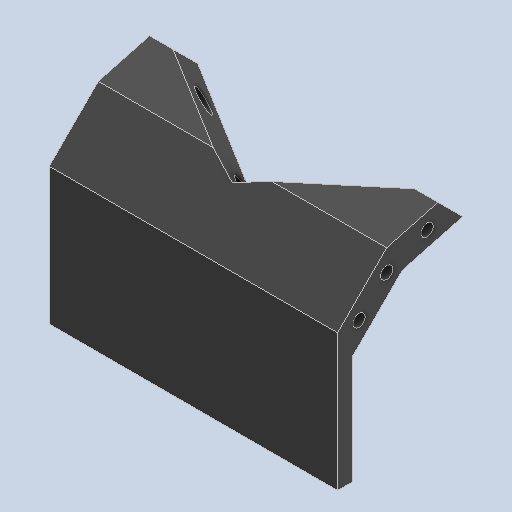
# Autodesk Inventor part: upper
Saved by Autodesk Inventor 2024.1 (Build 281209000, 209)
## iProperties
Created: 2024-10-11
Part Number: upper
Material: 一般
Document SubType Name: Modeling
Designer: hibik
Density: 1 g/cm^3
Appearance: 既定
Author: hibik
Autodesk Inventor part; units mm, degrees
ref_plane "YZ Plane" through (0, 0, 0) normal (1, 0, 0) x (0, 1, 0)
ref_plane "XZ Plane" through (0, 0, 0) normal (0, 1, 0) x (-1, 0, 0)
sketch "スケッチ1" plane through (0, 0, 0) normal (1, 0, 0) x (0, 1, 0)
  line L0 (0, 0) -> (18, 0)
  line L1 (18, 0) -> (18, -2)
  line L2 (18, -2) -> (0, -2)
  line L3 (0, -2) -> (0, 0)
  line L4 (18, 0) -> (39.2132, -21.2132)
  line L5 (39.2132, -21.2132) -> (37.799, -22.6274)
  line L6 (37.799, -22.6274) -> (17.1716, -2)
  dimension "d0" = 2
  dimension "d1" = 18
  dimension "d4" = 30
  dimension "d5" = 135
  dimension "d6" = 2
  constraints: 14 end point, 3 perpendicular, 2 parallel, 1 horizontal, 1 point on line
  measures "d0" distance of L0.end L1.end
  measures "d1" distance of L1.end L2.end
  measures "d4" distance from line of L0.end L5
  measures "d5" angle of L0 L4
  measures "d6" distance from line of L4.end L6
extrude "押し出し1" add sketch "スケッチ1" along normal blind 38
sketch "スケッチ2" plane through (38, 0, 0) normal (1, 0, 0) x (0, 0, -1)
  line L0 (13.2259, 26.2762) -> (6.4645, 24.4645) projected
  line L1 (2, 0) -> (2, 17.1716) projected
  line L2 (2, 17.1716) -> (22.6274, 37.799) projected
  line L3 (22.6274, 37.799) -> (21.2132, 39.2132) projected
  line L4 (21.2132, 39.2132) -> (0, 18) projected
  line L5 (0, 18) -> (0, 0) projected
  line L6 (0, 0) -> (2, 0) projected
  point P0 (10.3282, 25.4997)
extrude "押し出し2" cut sketch "スケッチ2" against normal through all contours L0 L4 L3 L2
sketch "スケッチ3" plane through (38, 0, 0) normal (1, 0, 0) x (0, 0, -1)
  line L0 (0, -0.1838) -> (49.5981, -49.7818) projected
  line L1 (49.5981, -49.7818) -> (50.9877, -48.3922) projected
  line L2 (50.9877, -48.3922) -> (50.3051, -40.5894) projected
  line L3 (50.3051, -40.5894) -> (38.2775, -28.5617) projected
  line L4 (38.2775, -28.5617) -> (34.3952, -14.0729) projected
  line L5 (34.3952, -14.0729) -> (39.6985, -8.7696) projected
  line L6 (25.2028, 5.7261) -> (39.6985, -8.7696) projected
  line L7 (25.2028, 9.9688) -> (25.2468, 10.0127) projected
  line L8 (25.2468, 14.2554) -> (13.2259, 26.2762) projected
  line L9 (13.2259, 26.2762) -> (6.4645, 24.4645) projected
  line L10 (6.4645, 24.4645) -> (0, 18) projected
  circle A0 centre (45.0018, -38.8216) radius 0.8 projected
  circle A1 centre (48.5373, -42.3571) radius 0.8 projected
  line L11 (25.2886, 2.8119) -> (28.6525, -0.552) projected
  arc A2 (29.0919, -1.6127) -> (28.6525, -0.552) centre (27.5919, -1.6127) ccw projected
  line L12 (29.0919, -1.6127) -> (29.0919, -20.7046) projected
  arc A3 (26.5312, -21.7652) -> (29.0919, -20.7046) centre (27.5919, -20.7046) ccw projected
  line L13 (26.5312, -21.7652) -> (23.1673, -18.4013) projected
  arc A4 (22.7279, -17.3406) -> (23.1673, -18.4013) centre (24.2279, -17.3406) ccw projected
  line L14 (22.7279, -17.3406) -> (22.7279, 1.7513) projected
  arc A5 (25.2886, 2.8119) -> (22.7279, 1.7513) centre (24.2279, 1.7513) ccw projected
  line L15 (13.8033, -9.0373) -> (10.4393, -5.6734) projected
  arc A6 (10, -4.6127) -> (10.4393, -5.6734) centre (11.5, -4.6127) ccw projected
  line L16 (10, -4.6127) -> (10, 14.4792) projected
  arc A7 (12.5607, 15.5398) -> (10, 14.4792) centre (11.5, 14.4792) ccw projected
  line L17 (12.5607, 15.5398) -> (15.9246, 12.1759) projected
  arc A8 (16.364, 11.1152) -> (15.9246, 12.1759) centre (14.864, 11.1152) ccw projected
  line L18 (16.364, 11.1152) -> (16.364, -7.9767) projected
  arc A9 (13.8033, -9.0373) -> (16.364, -7.9767) centre (14.864, -7.9767) ccw projected
  line L19 (2, 0) -> (2, 17.1716) projected
  line L20 (2, 14.3431) -> (13.5795, 25.9226)
  line L21 (16.4919, 23.0102) -> (8.535, 20.8782)
  line L22 (6.4645, 24.4645) -> (0, 18) projected
  line L23 (2, 17.1716) -> (10.3282, 25.4997) projected
  circle A10 centre (11.8117, 23.8267) radius 0.8 projected
  circle A11 centre (2.8284, 18) radius 0.8 projected
  circle A12 centre (6.4645, 21.636) radius 0.8 projected
  arc A13 (25.2028, 9.9688) -> (25.2028, 5.7261) centre (27.3241, 7.8475) ccw projected
  circle A14 centre (16.7615, 19.9122) radius 0.8 projected
  line L24 (0, 18) -> (0, -0.1838) projected
  arc A15 (25.2468, 10.0127) -> (25.2468, 14.2554) centre (23.1254, 12.1341) ccw projected
  circle A16 centre (20.297, 16.3767) radius 0.8 projected
  point P0 (0, 0)
  dimension "d9" = 4
  dimension "d10" = 4
  constraints: 4 end point, 4 point on line, 2 parallel, 1 perpendicular
  measures "d9" distance between parallel lines of L10 L20
  measures "d10" distance between parallel lines of L9 L21
ref_plane "作業平面1" through (0, -49.7818, -69.441) normal (1, 0, 0) x (0, 0.7071068, -0.7071068)
extrude "押し出し3" add sketch "スケッチ3" against normal up to surface (38 mm away) contours L9 L8 L20 A10 L19 L23 A11 A12 | A12 L23 | L8 L21 L20 A10 | A10 L20 | L20 A10 | A11 L23 picked at (6.7643, 21.5956) picked at (2.746, 17.7464)
sketch "スケッチ4" plane through (38, 0, 0) normal (1, 0, 0) x (0, 0, -1)
  circle A0 centre (2.8284, 18) radius 0.8
  circle A1 centre (6.4645, 21.636) radius 0.8
  circle A2 centre (11.8117, 23.8267) radius 0.8
  line L0 (6.4645, 24.4645) -> (0, 18) projected
  line L1 (13.2259, 26.2762) -> (6.4645, 24.4645) projected
  line L2 (11.8117, 23.8267) -> (11.2941, 25.7586)
  point P0 (0, 0)
  dimension "d13" = 1.6
  dimension "d14" = 2
  dimension "d15" = 2
  dimension "d16" = 2
  dimension "d17" = 2
  constraints: 3 centre point, 2 end point, 2 equal radius, 1 horizontal alignment, 1 perpendicular, 1 point on line, 1 vertical alignment
  measures "d13" diameter of A0
  measures "d14" distance from line of L0 A0.centre
  measures "d15" distance from line of L0 A1.centre
  measures "d16" distance from line of L1 L2.start
  measures "d17" distance from line of L1.start L2
extrude "押し出し4" cut sketch "スケッチ4" against normal through all
sketch "スケッチ5" plane through (0, 18, 0) normal (0, 0.7071068, 0.7071068) x (1, 0, 0)
  line L0 (19, 8.3282) -> (1.5, 17.1212) projected
  line L1 (36.5, 17.1212) -> (19, 8.3282) projected
  line L2 (38, 15.2043) -> (0, 15.2043) projected
  line L3 (3.0877, 15.2043) -> (19, 7.209)
  line L4 (38, 15.2043) -> (0, 15.2043) projected
  line L5 (34.9123, 15.2043) -> (19, 7.209)
  point P0 (0, -12.7279)
  dimension "d20" = 1
  constraints: 4 end point, 2 parallel, 2 point on line, 1 vertical alignment
  measures "d20" distance between parallel lines of L3 L0
extrude "押し出し5" cut sketch "スケッチ5" against normal through all
equation "\"d15\" = d14"
